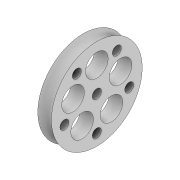
# Autodesk Inventor part: Pulley_18mm
Saved by Autodesk Inventor 2022 (Build 260153000, 153)
## iProperties
Created: 2022-07-09
Part Number: Pulley_18mm
Material: Generic
Document SubType Name: Modeling
Designer: dell
Density: 1 g/cm^3
Appearance: Default
Author: dell
Autodesk Inventor part; units mm, degrees
ref_plane "YZ Plane" through (0, 0, 0) normal (1, 0, 0) x (0, 1, 0)
ref_plane "XZ Plane" through (0, 0, 0) normal (0, 1, 0) x (-1, 0, 0)
ref_plane "XY Plane" through (0, 0, 0) normal (0, 0, 1) x (1, 0, 0)
sketch "Sketch1" plane through (0, 0, 0) normal (0, 0, 1) x (1, 0, 0)
  line L0 (-3, 0) -> (3, 0)
  line L1 (3, 0) -> (3, 20)
  line L2 (3, 20) -> (-3, 20)
  line L3 (-3, 20) -> (-3, 0)
  line L4 (-4.2, 0) -> (4.2, 0) projected
  arc A0 (-3, 20) -> (3, 20) centre (0, 21.3748) ccw
  point P0 (0, 0)
  dimension "d0" = 6
  dimension "d1" = 3
  dimension "d2" = 20
  dimension "d16" = 3.3
  constraints: 8 end point, 2 parallel, 2 point on circle, 1 centre point, 1 horizontal, 1 midpoint, 1 perpendicular
  measures "d0" distance between parallel lines of L3 L1
  measures "d1" distance from line of point (0, 0) L1
  measures "d2" distance between parallel lines of L2 L0
  measures "d16" radius of A0
revolve "Revolution1" add sketch "Sketch1" angle 360 about axis through (-10, 0, 0) along (1, 0, 0) contours L3 A0 L1 L0
sketch "Sketch2" plane through (3, 0, 0) normal (1, 0, 0) x (0, 0, -1)
  circle A0 centre (0, 0) radius 2.05
  dimension "d5" = 4.1
  constraints: 1 centre point, 1 coincident
  measures "d5" diameter of A0
extrude "Extrusion1" cut sketch "Sketch2" along normal mid plane 10
sketch "Sketch3" plane through (3, 0, 0) normal (1, 0, 0) x (0, 0, -1)
  circle A0 centre (0, 11) radius 5
  circle A1 centre (-8.8168, 12.1353) radius 2
  line L0 (-8.8168, 12.1353) -> (0, 0) construction
  line L1 (0, -28) -> (0, 28) construction
  dimension "d8" = 10
  dimension "d9" = 11
  dimension "d17" = 4
  dimension "d18" = 15
  dimension "d19" = 36
  constraints: 2 centre point, 2 end point
  measures "d8" diameter of A0
  measures "d9" distance of L0.end A0.centre
  measures "d17" diameter of A1
  measures "d18" distance of L0.end L0.start
  measures "d19" angle of L1 L0
extrude "Extrusion2" cut sketch "Sketch3" along normal mid plane 100
pattern_circular "Circular Pattern1" count 5 over 360 about axis through (-10, 0, 0) along (1, 0, 0) of "Extrusion2"
equation "\"d1\" = 0.5 * d0"
body "Solid1"
